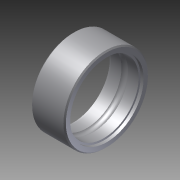
# Autodesk Inventor part: WML5010ZZ Outer ring
Saved by Autodesk Inventor 2013 SP2 (Build 170200200, 200)
## iProperties
Category: PARTsolutions
Company: KOYO
Created: 2013-06-21
Part Number: WML5010ZZ Outer ring
Catalog Web Link: www.cadenas.de
Description: Open Outer ring-
Vendor: KOYO
Document SubType Name: Modeling
Designer: PARTuser1
Manufacturer: KOYO
Density: 1 g/cm^3
Material: Generic
PSOL_IDENT_0: {$CADENAS_DATA\23d-libs\koyo\deep_groove_ball_bearings\extra_small_bb_miniature_bb\extra_small_bb_mi
PSOL_IDENT_1: niature_bb\open_or.prj},193 {VTYP=3D},{NB=WML5010ZZ Outer ring},{LINA=WML5010ZZ Outer ring},{NN=Open
PSOL_IDENT_2: Outer ring},{DATE=23.11.2007 06:29:51},{GEOMDATE=23.11.2007 00:00:00},{VERSION=},{LINEID=1000},{LIN
PSOL_IDENT_3: ESUBID=-1},{WBVAR=}  {NB=WML5010ZZ Outer ring},{LINA=WML5010ZZ Outer ring},{KT=DUMMY},{SRS=BS},{TP=6
PSOL_IDENT_4: 0},{SD=5.0},{D=10},{B=4.0},{R=0.10},{ORDER=WML5010ZZ},{VERS1=2.0},{VERS=2.000},{ST=2-D},{C=0.43},{C0
PSOL_IDENT_5: =0.17},{NG=55000},{NO=0},{SR=0.20},{DF1=0.0},{BF1=0.0},{BD=1.20},{PCD=7.35},{ID=6.45},{OD=8.25},{GID
PSOL_IDENT_6: =6.45},{GOD=8.70},{X1=0.36},{X2=0.15},{NOB=10}
CNS_NB: WML5010ZZ Outer ring
CNS_NBSYN: $ORDER. Outer ring
CNS_LINA: WML5010ZZ Outer ring
CNS_SRS: BS
CNS_TP: 60
CNS_SD: 5.0
CNS_D: 10
CNS_B: 4.0
CNS_R: 0.10
CNS_ORDER: WML5010ZZ
CNS_VERS1: 2.0
CNS_VERS: 2.000
CNS_ST: 2-D
CNS_C: 0.43
CNS_C0: 0.17
CNS_NG: 55000
CNS_NO: 0
CNS_SR: 0.20
CNS_DF1: 0.0
CNS_BF1: 0.0
CNS_BD: 1.20
CNS_PCD: 7.35
CNS_ID: 6.45
CNS_OD: 8.25
CNS_GID: 6.45
CNS_GOD: 8.70
CNS_X1: 0.36
CNS_X2: 0.15
CNS_NOB: 10
SUPPLIER: KOYO
ARTICLENO: WML5010ZZ Outer ring
BOMINFO: WML5010ZZ Outer ring
CREATOR: CADENAS GmbH
Title: WML5010ZZ Outer ring
Author: Cadenas PARTsolutions
Autodesk Inventor part; units mm, degrees
sketch "Sketch_4" plane through (0, 0, 0) normal (0, 0, 1) x (1, 0, 0)
  line L0 (4, 0) -> (0, 0)
  line L1 (0, 4.8586) -> (0, 4.35)
  line L2 (0, 4.35) -> (0.36, 4.35)
  line L3 (0.36, 4.35) -> (0.36, 4.125)
  line L4 (0.36, 4.125) -> (1.6031, 4.125)
  arc A0 (2.3969, 4.125) -> (1.6031, 4.125) centre (2, 3.675) ccw
  line L5 (2.3969, 4.125) -> (3.64, 4.125)
  line L6 (3.64, 4.125) -> (3.64, 4.35)
  line L7 (3.64, 4.35) -> (4, 4.35)
  line L8 (4, 4.35) -> (4, 4.8586)
  line L9 (4, 4.8586) -> (3.8586, 5)
  line L10 (3.8586, 5) -> (0.1414, 5)
  line L11 (0.1414, 5) -> (0, 4.8586)
  constraints: 24 end point, 2 point on circle, 1 centre point
revolve "Revolution1" add sketch "Sketch_4" angle 360 about axis through (4, 0, 0) along (1, 0, 0)
ref_plane "center_XY" through (0, 0, 0) normal (1, 0, 0) x (0, 0, -1)
ref_plane "center_YZ" through (0, 0, 0) normal (0, 0, -1) x (0, 1, 0)
ref_plane "center_ZX" through (0, 0, 0) normal (0, 1, 0) x (1, 0, 0)
ref_plane "or_1_1_XY" through (2, 3.675, 0) normal (1, 0, 0) x (0, 0, -1)
ref_plane "or_1_1_YZ" through (2, 3.675, 0) normal (0, 0, -1) x (0, 1, 0)
ref_plane "or_1_1_ZX" through (2, 3.675, 0) normal (0, 1, 0) x (1, 0, 0)
ref_plane "or_1_10_XY" through (2, 2.9731, -2.1601) normal (1, 0, 0) x (0, 0, -1)
ref_plane "or_1_10_YZ" through (2, 2.9731, -2.1601) normal (0, 0, -1) x (0, 1, 0)
ref_plane "or_1_10_ZX" through (2, 2.9731, -2.1601) normal (0, 1, 0) x (1, 0, 0)
ref_plane "or_1_2_XY" through (2, 2.9731, 2.1601) normal (1, 0, 0) x (0, 0, -1)
ref_plane "or_1_2_YZ" through (2, 2.9731, 2.1601) normal (0, 0, -1) x (0, 1, 0)
ref_plane "or_1_2_ZX" through (2, 2.9731, 2.1601) normal (0, 1, 0) x (1, 0, 0)
ref_plane "or_1_3_XY" through (2, 1.1356, 3.4951) normal (1, 0, 0) x (0, 0, -1)
ref_plane "or_1_3_YZ" through (2, 1.1356, 3.4951) normal (0, 0, -1) x (0, 1, 0)
ref_plane "or_1_3_ZX" through (2, 1.1356, 3.4951) normal (0, 1, 0) x (1, 0, 0)
ref_plane "or_1_4_XY" through (2, -1.1356, 3.4951) normal (1, 0, 0) x (0, 0, -1)
ref_plane "or_1_4_YZ" through (2, -1.1356, 3.4951) normal (0, 0, -1) x (0, 1, 0)
ref_plane "or_1_4_ZX" through (2, -1.1356, 3.4951) normal (0, 1, 0) x (1, 0, 0)
ref_plane "or_1_5_XY" through (2, -2.9731, 2.1601) normal (1, 0, 0) x (0, 0, -1)
ref_plane "or_1_5_YZ" through (2, -2.9731, 2.1601) normal (0, 0, -1) x (0, 1, 0)
ref_plane "or_1_5_ZX" through (2, -2.9731, 2.1601) normal (0, 1, 0) x (1, 0, 0)
ref_plane "or_1_6_XY" through (2, -3.675, 0) normal (1, 0, 0) x (0, 0, -1)
ref_plane "or_1_6_YZ" through (2, -3.675, 0) normal (0, 0, -1) x (0, 1, 0)
ref_plane "or_1_6_ZX" through (2, -3.675, 0) normal (0, 1, 0) x (1, 0, 0)
ref_plane "or_1_7_XY" through (2, -2.9731, -2.1601) normal (1, 0, 0) x (0, 0, -1)
ref_plane "or_1_7_YZ" through (2, -2.9731, -2.1601) normal (0, 0, -1) x (0, 1, 0)
ref_plane "or_1_7_ZX" through (2, -2.9731, -2.1601) normal (0, 1, 0) x (1, 0, 0)
ref_plane "or_1_8_XY" through (2, -1.1356, -3.4951) normal (1, 0, 0) x (0, 0, -1)
ref_plane "or_1_8_YZ" through (2, -1.1356, -3.4951) normal (0, 0, -1) x (0, 1, 0)
ref_plane "or_1_8_ZX" through (2, -1.1356, -3.4951) normal (0, 1, 0) x (1, 0, 0)
ref_plane "or_1_9_XY" through (2, 1.1356, -3.4951) normal (1, 0, 0) x (0, 0, -1)
ref_plane "or_1_9_YZ" through (2, 1.1356, -3.4951) normal (0, 0, -1) x (0, 1, 0)
ref_plane "or_1_9_ZX" through (2, 1.1356, -3.4951) normal (0, 1, 0) x (1, 0, 0)
ref_plane "outer_XY" through (4, 0, 0) normal (1, 0, 0) x (0, 0, -1)
ref_plane "outer_YZ" through (4, 0, 0) normal (0, 0, -1) x (0, 1, 0)
ref_plane "outer_ZX" through (4, 0, 0) normal (0, 1, 0) x (1, 0, 0)
body "Solid1"
